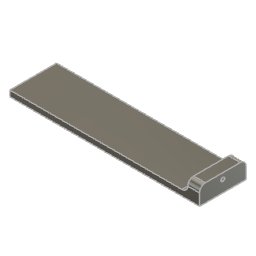
FinalCSProject5 v3 (Autodesk Fusion 360 design; units mm, degrees)
Autodesk Fusion 360 part; units mm, degrees
sketch "Sketch1" plane through (0, 0, 0) normal (0, 1, 0) x (1, 0, 0)
  line L0 (0, 0) -> (162.5, 0)
  line L1 (162.5, 0) -> (162.5, 40)
  line L2 (162.5, 40) -> (0, 40)
  line L3 (0, 40) -> (0, 0)
  dimension "d1" = 162.5
  dimension "d2" = 40
  constraint horizontal L0
  constraint vertical L1
  constraint horizontal L2
  constraint vertical L3
  constraint coincident L0.start L3.end
  measures "d1" distance of L0.start L0.end
  measures "d2" distance of L0.end L1.end
extrude "Extrude1" add sketch "Sketch1" along normal blind 5
sketch "Sketch2" plane through (0, 5, 0) normal (0, 1, 0) x (-1, 0, 0)
  line L0 (0, -40) -> (0, 0)
  line L1 (0, 0) -> (-162.5, 0)
  line L2 (-162.5, 0) -> (-162.5, -40)
  line L3 (-162.5, -40) -> (0, -40)
  line L4 (-162.5, -40) -> (-152.5, -40)
  line L5 (-152.5, -40) -> (-152.5, 0)
  line L6 (-152.5, 0) -> (-162.5, 0)
  line L7 (-162.5, 0) -> (-162.5, -40)
  dimension "d10" = 10
  constraint horizontal L4
  constraint vertical L5
  constraint horizontal L6
  constraint vertical L7
  constraint coincident L1 L5.end
  constraint coincident L2.end L3.start
  measures "d10" distance of L2.end L4.end
extrude "Extrude2" add sketch "Sketch2" along normal blind 10 contours L1 L2 L3 L4 L5 L6 L7
sketch "Sketch3" plane through (152.5, 0, 0) normal (-1, 0, 0) x (0, 0, 1)
  line L0 (-40, 5) -> (0, 5)
  line L1 (0, 5) -> (0, 15)
  line L2 (0, 15) -> (-40, 15)
  line L3 (-40, 15) -> (-40, 5)
  line L4 (-40, 15) -> (0, 5) construction
  line L5 (-40, 5) -> (0, 15) construction
  circle A0 centre (-20, 10) radius 1.6
  circle A1 centre (-20, 10) radius 2.85
  dimension "d7" = 3.2
  dimension "d15" = 5.7
  constraint coincident L2.end L3.start
  constraint coincident L0.end L1.start
  constraint coincident L0.start L3.end
  constraint coincident L1.end L2.start
  constraint midpoint L5 A0.centre
  constraint concentric A0 A1
  measures "d7" diameter of A0
  measures "d15" diameter of A1
extrude "Extrude3" cut sketch "Sketch3" against normal blind 10.5 contours A0
fillet "Fillet1" radius 5 1 edges at (157.5, 15, 0)
extrude "Extrude4" cut sketch "Sketch3" along normal blind -5 and the other way blind 0 contours A1
fillet "Fillet3" radius 5 1 edges at (152.5, 5, -20)
fillet "Fillet4" radius 5 1 edges at (157.5, 15, -40)
